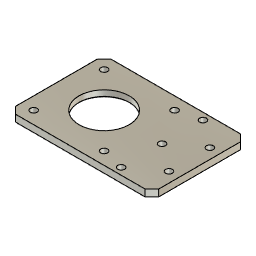
_机械臂组装 v14 (Autodesk Fusion 360 archive; units mm, degrees)
design "42电机输出固定"
Autodesk Fusion 360 part; units mm, degrees
(part 1 of 3)
sketch "草图1" plane through (0, 0, 0) normal (0, 0, 1) x (1, 0, 0)
  circle A0 centre (0, 0) radius 11.025
  line L0 (18, 21) -> (-18, 21)
  line L1 (-21, 18) -> (-21, -18)
  line L2 (-18, -21) -> (18, -21)
  line L3 (21, -18) -> (21, 18)
  line L4 (21, 21) -> (-21, -21) construction
  line L5 (-21, 21) -> (21, -21) construction
  circle A1 centre (15.5, -15.5) radius 1.5
  circle A2 centre (15.5, 15.5) radius 1.5
  circle A3 centre (-15.5, 15.5) radius 1.5
  circle A4 centre (-15.5, -15.5) radius 1.5
  line L6 (-18, 21) -> (-21, 18)
  line L7 (-21, -18) -> (-18, -21)
  line L8 (18, 21) -> (21, 18)
  line L9 (21, -18) -> (18, -21)
  line L10 (42, 18) -> (42, -18)
  line L11 (21, -18) -> (21, 18)
  line L12 (18, 21) -> (39, 21)
  line L13 (39, -21) -> (18, -21)
  circle A5 centre (25.5, 0) radius 1.5
  circle A6 centre (25.5, -18) radius 1.5
  circle A7 centre (37.5, -9) radius 1.5
  line L14 (79.2108, 0) -> (-40, 0) construction
  circle A8 centre (37.5, 9) radius 1.5
  circle A9 centre (25.5, 18) radius 1.5
  line L15 (39, 21) -> (42, 18)
  line L16 (42, -18) -> (39, -21)
  point P0 (42, 21)
  point P1 (42, -21)
  dimension "d1" = 22.05
  dimension "d2" = 42
  dimension "d3" = 42
  dimension "d4" = 15.5
  dimension "d5" = 3
  dimension "d7" = 360
  dimension "d8" = 3
  dimension "d9" = 3
  dimension "d10" = 3
  dimension "d11" = 3
  dimension "d12" = 3
  dimension "d13" = 3
  dimension "d14" = 3
  dimension "d15" = 3
  dimension "d17" = 21
  dimension "d20" = 3
  dimension "d21" = 3
  dimension "d22" = 3
  dimension "d24" = 18
  dimension "d25" = 9
  dimension "d26" = 4.5
  dimension "d27" = 4.5
  dimension "d28" = 16.5
  dimension "d30" = 3
  dimension "d31" = 3
  dimension "d32" = 3
  dimension "d33" = 3
  constraint coincident A0.centre origin
  constraint horizontal L0
  constraint perpendicular L0 L1
  constraint parallel L0 L2
  constraint parallel L1 L3
  constraint coincident L4 A0.centre
  constraint coincident L5 A0.centre
  constraint coincident L5 A1.centre
  constraint coincident L5.start L0
  constraint coincident L5.start L1
  constraint coincident L4.end L1
  constraint coincident L4.end L2
  constraint coincident L4.start L0
  constraint coincident L4.start L3
  constraint coincident L5.end L3
  constraint coincident L5.end L2
  constraint vertical L10
  constraint vertical L11
  constraint horizontal L12
  constraint horizontal L13
  constraint horizontal L14
  constraint coincident A0.centre L14
  constraint coincident A5.centre L14
  constraint symmetric A6 L14 A9
  constraint symmetric A7 L14 A8
  constraint coincident P0 L12
  constraint coincident P0 L10
  constraint coincident P1 L10
  constraint coincident P1 L13
  measures "d1" diameter of A0
  measures "d2" distance of L4.start L5.start
  measures "d3" distance of L4.start L5.end
  measures "d4" horizontal distance of A0.centre A1.centre
  measures "d5" diameter of A1
  measures "d8" distance of L5.start L0.end
  measures "d9" distance of L5.start L1.start
  measures "d10" distance of L4.end L1.end
  measures "d11" distance of L4.end L2.start
  measures "d12" distance of L4.start L0.start
  measures "d13" distance of L4.start L3.end
  measures "d14" distance of L5.end L3.start
  measures "d15" distance of L5.end L2.end
  measures "d17" distance of L10 L11
  measures "d20" diameter of A6
  measures "d21" diameter of A5
  measures "d22" diameter of A7
  measures "d24" distance of A6.centre L14
  measures "d25" distance of A7.centre L14
  measures "d26" distance of L11 A5.centre
  measures "d27" distance of L11 A6.centre
  measures "d28" distance of L3 A7.centre
  measures "d30" distance of P0 L12.end
  measures "d31" distance of P0 L10.start
  measures "d32" distance of P1 L10.end
  measures "d33" distance of P1 L13.start
extrude "拉伸1" add sketch "草图1" along normal blind 3
chamfer "倒角1" distance 0.5 angle 45 1 edges at (-10.2789, 3.9868, 0)
equation "d9 = d8"
equation "d11 = d10"
equation "d13 = d12"
equation "d15 = d14"
equation "d31 = d30"
equation "d33 = d32"

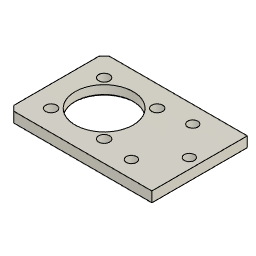
design "28减速输出固定"
Autodesk Fusion 360 part; units mm, degrees
sketch "草图4" plane through (0, 0, 0) normal (0, 0, 1) x (1, 0, 0)
  line L0 (12.5, 14) -> (-12.5, 14)
  line L1 (-14, 12.5) -> (-14, -12.5)
  line L2 (-12.5, -14) -> (12.5, -14)
  line L3 (14, -12.5) -> (14, 12.5)
  line L4 (14, 14) -> (-14, -14) construction
  line L5 (-14, 14) -> (14, -14) construction
  line L6 (12.5, 14) -> (14, 12.5)
  line L7 (14, -12.5) -> (12.5, -14)
  line L8 (-12.5, -14) -> (-14, -12.5)
  line L9 (-14, 12.5) -> (-12.5, 14)
  circle A0 centre (7.7782, 7.7782) radius 1.609
  circle A1 centre (0, 0) radius 8.5
  circle A2 centre (-7.7782, 7.7782) radius 1.609
  circle A3 centre (-7.7782, -7.7782) radius 1.609
  circle A4 centre (7.7782, -7.7782) radius 1.609
  line L10 (0, -35) -> (0, 45.3825) construction
  line L11 (12.5, 14) -> (28, 14)
  line L12 (28, 14) -> (28, -14)
  line L13 (28, -14) -> (12.5, -14)
  line L14 (-31, 0) -> (62, 0) construction
  circle A5 centre (25, 0) radius 1.5
  circle A6 centre (17, -9) radius 1.5
  circle A7 centre (17, 9) radius 1.5
  dimension "d49" = 28
  dimension "d50" = 28
  dimension "d51" = 1.5
  dimension "d52" = 1.5
  dimension "d53" = 1.5
  dimension "d54" = 1.5
  dimension "d55" = 1.5
  dimension "d56" = 1.5
  dimension "d57" = 1.5
  dimension "d58" = 1.5
  dimension "d59" = 11
  dimension "d60" = 17
  dimension "d62" = 360
  dimension "d71" = 14
  dimension "d72" = 3
  dimension "d73" = 3
  dimension "d74" = 3
  dimension "d75" = 11
  dimension "d76" = 9
  constraint horizontal L0
  constraint perpendicular L0 L1
  constraint parallel L0 L2
  constraint parallel L1 L3
  constraint coincident L4 A1.centre
  constraint coincident L5 A1.centre
  constraint coincident A1.centre origin
  constraint coincident L4.start L0
  constraint coincident L4.start L3
  constraint coincident L5.end L3
  constraint coincident L5.end L2
  constraint coincident L4.end L2
  constraint coincident L4.end L1
  constraint coincident L5.start L1
  constraint coincident L5.start L0
  constraint coincident L4 A0.centre
  constraint vertical L10
  constraint coincident A1.centre L10
  constraint parallel L0 L11
  constraint perpendicular L0 L12
  constraint horizontal L13
  constraint horizontal L14
  constraint coincident A1.centre L14
  constraint coincident L14 A5.centre
  constraint symmetric L14 A6 A7
  measures "d49" distance of L4.start L5.start
  measures "d50" distance of L5.start L4.end
  measures "d51" distance of L4.start L0.start
  measures "d52" distance of L4.start L3.end
  measures "d53" distance of L5.end L3.start
  measures "d54" distance of L5.end L2.end
  measures "d55" distance of L4.end L2.start
  measures "d56" distance of L4.end L1.end
  measures "d57" distance of L5.start L1.start
  measures "d58" distance of L5.start L0.end
  measures "d59" distance of A1.centre A0.centre
  measures "d60" diameter of A1
  measures "d71" distance of L3 L12
  measures "d72" diameter of A6
  measures "d73" diameter of A5
  measures "d74" distance of L3 A6.centre
  measures "d75" distance of L3 A5.centre
  measures "d76" distance of L14 A6.centre
extrude "拉伸3" add sketch "草图4" along normal blind 3
chamfer "倒角2" distance 0.5 angle 45 1 edges at (-7.9248, 3.0737, 0)
equation "d52 = d51"
equation "d54 = d53"
equation "d56 = d55"
equation "d58 = d57"

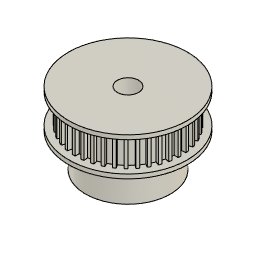
design "2GT40同步轮"
Autodesk Fusion 360 part; units mm, degrees
sketch "草图1" plane through (0, 0, 0) normal (0, 0, 1) x (1, 0, 0)
  circle A0 centre (0, 0) radius 10
  circle A1 centre (0, 0) radius 2.5
  dimension "d1" = 20
  dimension "d2" = 5
  constraint coincident A0.centre A1.centre
  measures "d1" diameter of A0
  measures "d2" diameter of A1
extrude "拉伸1" add sketch "草图1" along normal blind 8
sketch "草图2" plane through (0, 0, 0) normal (0, 0, 1) x (1, 0, 0)
  circle A0 centre (0, 0) radius 14
  line L0 (0, 0) -> (1.9515, 12.3214) construction
  line L1 (0, 0) -> (0, 12.475) construction
  line L2 (1.9501, 12.3124) -> (1.799, 11.3584)
  line L3 (1.799, 11.3584) -> (0.6019, 11.4842)
  line L4 (0.6529, 12.4579) -> (0, 12.4659)
  line L5 (0.6529, 12.4579) -> (0, 0) construction
  line L6 (0.6529, 12.4579) -> (0.6019, 11.4842)
  line L7 (0.6529, 12.4579) -> (0.6019, 11.4842)
  line L8 (-1.304, 12.4067) -> (-1.9501, 12.3124)
  line L9 (-1.304, 12.4067) -> (-1.2021, 11.437)
  line L10 (0, 11.5) -> (-1.2021, 11.437)
  line L11 (0, 12.4659) -> (0, 11.5)
  line L12 (-3.2288, 12.0499) -> (-3.8522, 11.8557)
  line L13 (-3.2288, 12.0499) -> (-2.9764, 11.1081)
  line L14 (-1.799, 11.3584) -> (-2.9764, 11.1081)
  line L15 (-1.9501, 12.3124) -> (-1.799, 11.3584)
  line L16 (-5.074, 11.3965) -> (-5.6594, 11.1072)
  line L17 (-5.074, 11.3965) -> (-4.6775, 10.5058)
  line L18 (-3.5537, 10.9371) -> (-4.6775, 10.5058)
  line L19 (-3.8522, 11.8557) -> (-3.5537, 10.9371)
  line L20 (-6.7944, 10.4624) -> (-7.3272, 10.0851)
  line L21 (-6.7944, 10.4624) -> (-6.2633, 9.6447)
  line L22 (-5.2209, 10.2466) -> (-6.2633, 9.6447)
  line L23 (-5.6594, 11.1072) -> (-5.2209, 10.2466)
  line L24 (-8.3474, 9.2707) -> (-8.8147, 8.8147)
  line L25 (-8.3474, 9.2707) -> (-7.695, 8.5462)
  line L26 (-6.7595, 9.3037) -> (-7.695, 8.5462)
  line L27 (-7.3272, 10.0851) -> (-6.7595, 9.3037)
  line L28 (-9.6949, 7.8508) -> (-10.0851, 7.3272)
  line L29 (-9.6949, 7.8508) -> (-8.9372, 7.2372)
  line L30 (-8.1317, 8.1317) -> (-8.9372, 7.2372)
  line L31 (-8.8147, 8.8147) -> (-8.1317, 8.1317)
  line L32 (-10.8037, 6.2375) -> (-11.1072, 5.6594)
  line L33 (-10.8037, 6.2375) -> (-9.9593, 5.75)
  line L34 (-9.3037, 6.7595) -> (-9.9593, 5.75)
  line L35 (-10.0851, 7.3272) -> (-9.3037, 6.7595)
  line L36 (-11.6464, 4.4706) -> (-11.8557, 3.8522)
  line L37 (-11.6464, 4.4706) -> (-10.7362, 4.1212)
  line L38 (-10.2466, 5.2209) -> (-10.7362, 4.1212)
  line L39 (-11.1072, 5.6594) -> (-10.2466, 5.2209)
  line L40 (-12.2024, 2.5937) -> (-12.3124, 1.9501)
  line L41 (-12.2024, 2.5937) -> (-11.2487, 2.391)
  line L42 (-10.9371, 3.5537) -> (-11.2487, 2.391)
  line L43 (-11.8557, 3.8522) -> (-10.9371, 3.5537)
  line L44 (-12.4579, 0.6529) -> (-12.4659, 0)
  line L45 (-12.4579, 0.6529) -> (-11.4842, 0.6019)
  line L46 (-11.3584, 1.799) -> (-11.4842, 0.6019)
  line L47 (-12.3124, 1.9501) -> (-11.3584, 1.799)
  line L48 (-12.4067, -1.304) -> (-12.3124, -1.9501)
  line L49 (-12.4067, -1.304) -> (-11.437, -1.2021)
  line L50 (-11.5, 0) -> (-11.437, -1.2021)
  line L51 (-12.4659, 0) -> (-11.5, 0)
  line L52 (-12.0499, -3.2288) -> (-11.8557, -3.8522)
  line L53 (-12.0499, -3.2288) -> (-11.1081, -2.9764)
  line L54 (-11.3584, -1.799) -> (-11.1081, -2.9764)
  line L55 (-12.3124, -1.9501) -> (-11.3584, -1.799)
  line L56 (-11.3965, -5.074) -> (-11.1072, -5.6594)
  line L57 (-11.3965, -5.074) -> (-10.5058, -4.6775)
  line L58 (-10.9371, -3.5537) -> (-10.5058, -4.6775)
  line L59 (-11.8557, -3.8522) -> (-10.9371, -3.5537)
  line L60 (-10.4624, -6.7944) -> (-10.0851, -7.3272)
  line L61 (-10.4624, -6.7944) -> (-9.6447, -6.2633)
  line L62 (-10.2466, -5.2209) -> (-9.6447, -6.2633)
  line L63 (-11.1072, -5.6594) -> (-10.2466, -5.2209)
  line L64 (-9.2707, -8.3474) -> (-8.8147, -8.8147)
  line L65 (-9.2707, -8.3474) -> (-8.5462, -7.695)
  line L66 (-9.3037, -6.7595) -> (-8.5462, -7.695)
  line L67 (-10.0851, -7.3272) -> (-9.3037, -6.7595)
  line L68 (-7.8508, -9.6949) -> (-7.3272, -10.0851)
  line L69 (-7.8508, -9.6949) -> (-7.2372, -8.9372)
  line L70 (-8.1317, -8.1317) -> (-7.2372, -8.9372)
  line L71 (-8.8147, -8.8147) -> (-8.1317, -8.1317)
  line L72 (-6.2375, -10.8037) -> (-5.6594, -11.1072)
  line L73 (-6.2375, -10.8037) -> (-5.75, -9.9593)
  line L74 (-6.7595, -9.3037) -> (-5.75, -9.9593)
  line L75 (-7.3272, -10.0851) -> (-6.7595, -9.3037)
  line L76 (-4.4706, -11.6464) -> (-3.8522, -11.8557)
  line L77 (-4.4706, -11.6464) -> (-4.1212, -10.7362)
  line L78 (-5.2209, -10.2466) -> (-4.1212, -10.7362)
  line L79 (-5.6594, -11.1072) -> (-5.2209, -10.2466)
  line L80 (-2.5937, -12.2024) -> (-1.9501, -12.3124)
  line L81 (-2.5937, -12.2024) -> (-2.391, -11.2487)
  line L82 (-3.5537, -10.9371) -> (-2.391, -11.2487)
  line L83 (-3.8522, -11.8557) -> (-3.5537, -10.9371)
  line L84 (-0.6529, -12.4579) -> (0, -12.4659)
  line L85 (-0.6529, -12.4579) -> (-0.6019, -11.4842)
  line L86 (-1.799, -11.3584) -> (-0.6019, -11.4842)
  line L87 (-1.9501, -12.3124) -> (-1.799, -11.3584)
  line L88 (1.304, -12.4067) -> (1.9501, -12.3124)
  line L89 (1.304, -12.4067) -> (1.2021, -11.437)
  line L90 (0, -11.5) -> (1.2021, -11.437)
  line L91 (0, -12.4659) -> (0, -11.5)
  line L92 (3.2288, -12.0499) -> (3.8522, -11.8557)
  line L93 (3.2288, -12.0499) -> (2.9764, -11.1081)
  line L94 (1.799, -11.3584) -> (2.9764, -11.1081)
  line L95 (1.9501, -12.3124) -> (1.799, -11.3584)
  line L96 (5.074, -11.3965) -> (5.6594, -11.1072)
  line L97 (5.074, -11.3965) -> (4.6775, -10.5058)
  line L98 (3.5537, -10.9371) -> (4.6775, -10.5058)
  line L99 (3.8522, -11.8557) -> (3.5537, -10.9371)
  line L100 (6.7944, -10.4624) -> (7.3272, -10.0851)
  line L101 (6.7944, -10.4624) -> (6.2633, -9.6447)
  line L102 (5.2209, -10.2466) -> (6.2633, -9.6447)
  line L103 (5.6594, -11.1072) -> (5.2209, -10.2466)
  line L104 (8.3474, -9.2707) -> (8.8147, -8.8147)
  line L105 (8.3474, -9.2707) -> (7.695, -8.5462)
  line L106 (6.7595, -9.3037) -> (7.695, -8.5462)
  line L107 (7.3272, -10.0851) -> (6.7595, -9.3037)
  line L108 (9.6949, -7.8508) -> (10.0851, -7.3272)
  line L109 (9.6949, -7.8508) -> (8.9372, -7.2372)
  line L110 (8.1317, -8.1317) -> (8.9372, -7.2372)
  line L111 (8.8147, -8.8147) -> (8.1317, -8.1317)
  line L112 (10.8037, -6.2375) -> (11.1072, -5.6594)
  line L113 (10.8037, -6.2375) -> (9.9593, -5.75)
  line L114 (9.3037, -6.7595) -> (9.9593, -5.75)
  line L115 (10.0851, -7.3272) -> (9.3037, -6.7595)
  line L116 (11.6464, -4.4706) -> (11.8557, -3.8522)
  line L117 (11.6464, -4.4706) -> (10.7362, -4.1212)
  line L118 (10.2466, -5.2209) -> (10.7362, -4.1212)
  line L119 (11.1072, -5.6594) -> (10.2466, -5.2209)
  line L120 (12.2024, -2.5937) -> (12.3124, -1.9501)
  line L121 (12.2024, -2.5937) -> (11.2487, -2.391)
  line L122 (10.9371, -3.5537) -> (11.2487, -2.391)
  line L123 (11.8557, -3.8522) -> (10.9371, -3.5537)
  line L124 (12.4579, -0.6529) -> (12.4659, 0)
  line L125 (12.4579, -0.6529) -> (11.4842, -0.6019)
  line L126 (11.3584, -1.799) -> (11.4842, -0.6019)
  line L127 (12.3124, -1.9501) -> (11.3584, -1.799)
  line L128 (12.4067, 1.304) -> (12.3124, 1.9501)
  line L129 (12.4067, 1.304) -> (11.437, 1.2021)
  line L130 (11.5, 0) -> (11.437, 1.2021)
  line L131 (12.4659, 0) -> (11.5, 0)
  line L132 (12.0499, 3.2288) -> (11.8557, 3.8522)
  line L133 (12.0499, 3.2288) -> (11.1081, 2.9764)
  line L134 (11.3584, 1.799) -> (11.1081, 2.9764)
  line L135 (12.3124, 1.9501) -> (11.3584, 1.799)
  line L136 (11.3965, 5.074) -> (11.1072, 5.6594)
  line L137 (11.3965, 5.074) -> (10.5058, 4.6775)
  line L138 (10.9371, 3.5537) -> (10.5058, 4.6775)
  line L139 (11.8557, 3.8522) -> (10.9371, 3.5537)
  line L140 (10.4624, 6.7944) -> (10.0851, 7.3272)
  line L141 (10.4624, 6.7944) -> (9.6447, 6.2633)
  line L142 (10.2466, 5.2209) -> (9.6447, 6.2633)
  line L143 (11.1072, 5.6594) -> (10.2466, 5.2209)
  line L144 (9.2707, 8.3474) -> (8.8147, 8.8147)
  line L145 (9.2707, 8.3474) -> (8.5462, 7.695)
  line L146 (9.3037, 6.7595) -> (8.5462, 7.695)
  line L147 (10.0851, 7.3272) -> (9.3037, 6.7595)
  line L148 (7.8508, 9.6949) -> (7.3272, 10.0851)
  line L149 (7.8508, 9.6949) -> (7.2372, 8.9372)
  line L150 (8.1317, 8.1317) -> (7.2372, 8.9372)
  line L151 (8.8147, 8.8147) -> (8.1317, 8.1317)
  line L152 (6.2375, 10.8037) -> (5.6594, 11.1072)
  line L153 (6.2375, 10.8037) -> (5.75, 9.9593)
  line L154 (6.7595, 9.3037) -> (5.75, 9.9593)
  line L155 (7.3272, 10.0851) -> (6.7595, 9.3037)
  line L156 (4.4706, 11.6464) -> (3.8522, 11.8557)
  line L157 (4.4706, 11.6464) -> (4.1212, 10.7362)
  line L158 (5.2209, 10.2466) -> (4.1212, 10.7362)
  line L159 (5.6594, 11.1072) -> (5.2209, 10.2466)
  line L160 (2.5937, 12.2024) -> (1.9501, 12.3124)
  line L161 (2.5937, 12.2024) -> (2.391, 11.2487)
  line L162 (3.5537, 10.9371) -> (2.391, 11.2487)
  line L163 (3.8522, 11.8557) -> (3.5537, 10.9371)
  circle A1 centre (0, 0) radius 2.5
  dimension "d5" = 28
  dimension "d6" = 9
  dimension "d7" = 12.475
  dimension "d12" = 360
  dimension "d16" = 11.5
  dimension "d17" = 11.5
  dimension "d19" = 3
  dimension "d23" = 5
  constraint coincident A0.centre L0.start
  constraint vertical L1
  constraint coincident L0 L2.end
  constraint parallel L0 L2
  constraint coincident L5 L3.end
  constraint equal L1 L5
  constraint equal L0 L1
  measures "d5" diameter of A0
  measures "d6" angle of L0 L1
  measures "d7" distance of A0.centre L1.end
  measures "d16" distance of A0.centre L3.end
  measures "d17" distance of A0.centre L2.end
  measures "d19" angle of L1 L6
  measures "d23" diameter of A1
extrude "拉伸2" add sketch "草图2" along normal blind 9 from surface at 8 contours A0 | L2 L3 L4 L6 L7 L8 L9 L10 L11 L12 L13 L14 L15 L16 L17 L18 L19 L20 L21 L22 L23 L24 L25 L26 L27 L28 L29 L30 L31 L32 L33 L34 L35 L36 L37 L38 L39 L40 L41 L42 L43 L44 L45 L46 L47 L48 L49 L50 L51 L52 L53 L54 L55 L56 L57 L58 L59 L60 L61 L62 L63 L64 L65 L66 L67 L68 L69 L70 L71 L72 L73 L74 L75 L76 L77 L78 L79 L80 L81 L82 L83 L84 L85 L86 L87 L88 L89 L90 L91 L92 L93 L94 L95 L96 L97 L98 L99 L100 L101 L102 L103 L104 L105 L106 L107 L108 L109 L110 L111 L112 L113 L114 L115 L116 L117 L118 L119 L120 L121 L122 L123 L124 L125 L126 L127 L128 L129 L130 L131 L132 L133 L134 L135 L136 L137 L138 L139 L140 L141 L142 L143 L144 L145 L146 L147 L148 L149 L150 L151 L152 L153 L154 L155 L156 L157 L158 L159 L160 L161 L162 L163
extrude "拉伸3" cut sketch "草图2" along normal blind 7 from surface at 9 contours A0

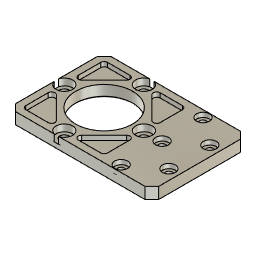
design "42减速输出固定"
Autodesk Fusion 360 part; units mm, degrees
sketch "草图1" plane through (0, 0, 0) normal (0, 0, 1) x (1, 0, 0)
  circle A0 centre (0, 0) radius 12.525
  line L0 (18, 21) -> (-18, 21)
  line L1 (-21, 18) -> (-21, -18)
  line L2 (-18, -21) -> (18, -21)
  line L3 (21, -18) -> (21, 18)
  line L4 (21, 21) -> (-21, -21) construction
  line L5 (-21, 21) -> (21, -21) construction
  line L6 (-18, 21) -> (-21, 18)
  line L7 (-21, -18) -> (-18, -21)
  line L8 (18, -21) -> (21, -18)
  line L9 (21, 18) -> (18, 21)
  line L10 (18, 21) -> (39, 21)
  line L11 (42, 18) -> (42, -18)
  line L12 (39, -21) -> (18, -21)
  circle A1 centre (0, 17.5) radius 2
  line L13 (0, 43) -> (0, -30.7766) construction
  circle A2 centre (-17.5, 0) radius 2
  circle A3 centre (0, -17.5) radius 2
  circle A4 centre (17.5, 0) radius 2
  circle A5 centre (37.5, 9) radius 1.5
  circle A6 centre (25.5, 0) radius 1.5
  circle A7 centre (37.5, -9) radius 1.5
  circle A8 centre (25.5, -18) radius 1.5
  circle A9 centre (25.5, 18) radius 1.5
  line L14 (-27.6866, 0) -> (52.7849, 0) construction
  line L15 (39, 21) -> (42, 18)
  line L16 (42, -18) -> (39, -21)
  point P0 (42, 21)
  point P1 (42, -21)
  dimension "d1" = 25.05
  dimension "d2" = 42
  dimension "d3" = 42
  dimension "d4" = 3
  dimension "d5" = 3
  dimension "d6" = 3
  dimension "d7" = 3
  dimension "d8" = 3
  dimension "d9" = 3
  dimension "d10" = 3
  dimension "d11" = 3
  dimension "d12" = 21
  dimension "d13" = 4
  dimension "d14" = 17.5
  dimension "d16" = 360
  dimension "d20" = 3
  dimension "d21" = 3
  dimension "d22" = 3
  dimension "d23" = 4.5
  dimension "d24" = 16.5
  dimension "d25" = 18
  dimension "d26" = 9
  dimension "d28" = 4.5
  dimension "d49" = 3
  dimension "d50" = 3
  dimension "d51" = 3
  dimension "d52" = 3
  constraint coincident A0.centre origin
  constraint horizontal L0
  constraint perpendicular L0 L1
  constraint parallel L0 L2
  constraint parallel L1 L3
  constraint coincident L4 A0.centre
  constraint coincident L5 A0.centre
  constraint coincident L5.start L0
  constraint coincident L5.start L1
  constraint coincident L4.end L1
  constraint coincident L4.end L2
  constraint coincident L5.end L2
  constraint coincident L5.end L3
  constraint coincident L4.start L3
  constraint coincident L4.start L0
  constraint parallel L0 L10
  constraint perpendicular L10 L11
  constraint perpendicular L2 L13
  constraint coincident A0.centre L13
  constraint coincident A1.centre L13
  constraint horizontal L14
  constraint coincident A0.centre L14
  constraint coincident A6.centre L14
  constraint symmetric A8 A9 L14
  constraint symmetric A5 A7 L14
  constraint horizontal L12
  constraint coincident P0 L10
  constraint coincident P0 L11
  constraint coincident P1 L11
  constraint coincident P1 L12
  measures "d1" diameter of A0
  measures "d2" distance of L4.start L5.end
  measures "d3" distance of L4.start L5.start
  measures "d4" distance of L5.start L0.end
  measures "d5" distance of L5.start L1.start
  measures "d6" distance of L4.end L1.end
  measures "d7" distance of L4.end L2.start
  measures "d8" distance of L5.end L2.end
  measures "d9" distance of L5.end L3.start
  measures "d10" distance of L4.start L3.end
  measures "d11" distance of L4.start L0.start
  measures "d12" distance of L3 L11
  measures "d13" diameter of A1
  measures "d14" distance of A0.centre A1.centre
  measures "d20" diameter of A8
  measures "d21" diameter of A6
  measures "d22" diameter of A7
  measures "d23" distance of L3 A6.centre
  measures "d24" distance of L3 A7.centre
  measures "d25" distance of A8.centre L14
  measures "d26" distance of A7.centre L14
  measures "d28" distance of L3 A8.centre
  measures "d49" distance of P0 L10.end
  measures "d50" distance of P0 L11.start
  measures "d51" distance of P1 L11.end
  measures "d52" distance of P1 L12.start
extrude "拉伸1" add sketch "草图1" along normal blind 5
sketch "草图2" plane through (0, 0, 5) normal (0, 0, 1) x (-1, 0, 0)
  circle A0 centre (-17.5, 0) radius 2
  circle A1 centre (0, -17.5) radius 2
  circle A2 centre (17.5, 0) radius 2
  circle A3 centre (0, 17.5) radius 2
  circle A4 centre (0, 0) radius 12.525
  circle A5 centre (-37.5, -9) radius 1.5
  circle A6 centre (-25.5, 0) radius 1.5
  circle A7 centre (-37.5, 9) radius 1.5
  circle A8 centre (-25.5, 18) radius 1.5
  circle A9 centre (-25.5, -18) radius 1.5
  line L0 (-39, -21) -> (18, -21)
  line L1 (18, -21) -> (21, -18)
  line L2 (21, -18) -> (21, 18)
  line L3 (21, 18) -> (18, 21)
  line L4 (18, 21) -> (-39, 21)
  line L5 (-42, 18) -> (-42, -18)
  circle A10 centre (0, -17.5) radius 2
  circle A11 centre (-25.5, 0) radius 1.5
  circle A12 centre (-37.5, -9) radius 1.5
  circle A13 centre (-25.5, -18) radius 1.5
  circle A14 centre (-37.5, 9) radius 1.5
  circle A15 centre (-25.5, 18) radius 1.5
  circle A16 centre (0, 17.5) radius 2
  circle A17 centre (-17.5, 0) radius 2
  circle A18 centre (17.5, 0) radius 2
  line L6 (-39, 21) -> (-42, 18)
  line L7 (-42, -18) -> (-39, -21)
  constraint concentric A1 A10
  constraint concentric A6 A11
  constraint concentric A5 A12
  constraint concentric A9 A13
  constraint concentric A7 A14
  constraint concentric A8 A15
  constraint concentric A3 A16
  constraint concentric A0 A17
  constraint concentric A2 A18
hole "孔1" at (-17.5, 0, 5) at (0, 17.5, 5) at (17.5, 0, 5) at (0, -17.5, 5) direction (0, 0, -1) diameter 4 depth 13 tip angle 180 counterbore diameter 7.25 counterbore depth 3
hole "孔2" at (25.5, 0, 5) at (37.5, 9, 5) at (25.5, 18, 5) at (37.5, -9, 5) at (25.5, -18, 5) direction (0, 0, -1) diameter 3 depth 13 tip angle 180 counterbore diameter 5.7 counterbore depth 2
chamfer "倒角1" distance 0.5 angle 45 1 edges at (-11.6774, 4.5292, 0)
sketch "草图3" plane through (0, 0, 0) normal (0, 0, 1) x (1, 0, 0)
  line L0 (-16.5, 18) -> (-6.6213, 18)
  line L1 (-5.5607, 15.4393) -> (-15.4393, 5.5607)
  line L2 (-18, 6.6213) -> (-18, 16.5)
  arc A0 (-5.5607, 15.4393) -> (-6.6213, 18) centre (-6.6213, 16.5) ccw
  arc A1 (-18, 6.6213) -> (-15.4393, 5.5607) centre (-16.5, 6.6213) ccw
  arc A2 (-16.5, 18) -> (-18, 16.5) centre (-16.5, 16.5) ccw
  line L3 (-18, -16.5) -> (-18, -6.6213)
  arc A3 (-15.4393, -5.5607) -> (-18, -6.6213) centre (-16.5, -6.6213) ccw
  line L4 (-15.4393, -5.5607) -> (-5.5607, -15.4393)
  arc A4 (-6.6213, -18) -> (-5.5607, -15.4393) centre (-6.6213, -16.5) ccw
  line L5 (-6.6213, -18) -> (-16.5, -18)
  arc A5 (-18, -16.5) -> (-16.5, -18) centre (-16.5, -16.5) ccw
  line L6 (16.5, -18) -> (6.6213, -18)
  arc A6 (5.5607, -15.4393) -> (6.6213, -18) centre (6.6213, -16.5) ccw
  line L7 (5.5607, -15.4393) -> (15.4393, -5.5607)
  arc A7 (18, -6.6213) -> (15.4393, -5.5607) centre (16.5, -6.6213) ccw
  line L8 (18, -6.6213) -> (18, -16.5)
  arc A8 (16.5, -18) -> (18, -16.5) centre (16.5, -16.5) ccw
  line L9 (18, 16.5) -> (18, 6.6213)
  arc A9 (15.4393, 5.5607) -> (18, 6.6213) centre (16.5, 6.6213) ccw
  line L10 (15.4393, 5.5607) -> (5.5607, 15.4393)
  arc A10 (6.6213, 18) -> (5.5607, 15.4393) centre (6.6213, 16.5) ccw
  line L11 (6.6213, 18) -> (16.5, 18)
  arc A11 (18, 16.5) -> (16.5, 18) centre (16.5, 16.5) ccw
  point P0 (-18, 18)
  point P1 (-3, 18)
  dimension "d40" = 18
  dimension "d41" = 18
  dimension "d42" = 15
  dimension "d43" = 1.5
  dimension "d45" = 360
  constraint horizontal L0
  constraint vertical L2
  constraint coincident P1 L0
  constraint coincident P1 L1
  constraint tangent L0 A0
  constraint tangent L1 A0
  constraint tangent L1 A1
  constraint tangent L2 A1
  constraint equal A0 A1
  constraint coincident P0 L2
  constraint coincident P0 L0
  constraint tangent L2 A2
  constraint tangent L0 A2
  constraint equal A0 A2
  constraint equal L0 L2
  measures "d40" distance of origin L0
  measures "d41" distance of origin L2
  measures "d42" distance of P0 P1
  measures "d43" radius of A0
extrude "拉伸2" cut sketch "草图3" against normal blind 2 from surface at 5
equation "d5 = d4"
equation "d7 = d6"
equation "d9 = d8"
equation "d11 = d10"
equation "d50 = d49"
equation "d52 = d51"

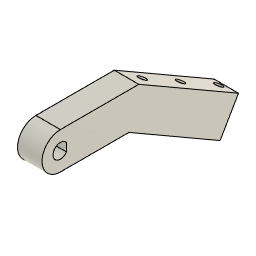
design "28输出Joint-4"
Autodesk Fusion 360 part; units mm, degrees
sketch "草图1" plane through (0, 0, 0) normal (1, 0, 0) x (0, 1, 0)
  circle A0 centre (0, 0) radius 7.5
  line L0 (0, 7.5) -> (32.0096, 7.5)
  line L1 (32.0096, 7.5) -> (72.7211, -16.0048)
  line L2 (72.7211, -16.0048) -> (65.2211, -28.9952)
  line L3 (65.2211, -28.9952) -> (27.9904, -7.5)
  line L4 (27.9904, -7.5) -> (0, -7.5)
  line L5 (0, 0) -> (30, 0) construction
  line L6 (30, 0) -> (68.9711, -22.5) construction
  line L7 (2.5, 1.6583) -> (2.5, -1.6583)
  arc A1 (2.5, 1.6583) -> (2.5, -1.6583) centre (0, 0) ccw
  dimension "d1" = 6
  dimension "d2" = 15
  dimension "d4" = 15
  dimension "d5" = 150
  dimension "d7" = 45
  dimension "d8" = 30
  dimension "d11" = 2.5
  constraint coincident A0.centre L5.start
  constraint concentric A0 A1
  constraint coincident A0 L0.start
  constraint tangent A0 L0
  constraint horizontal L0
  constraint parallel L1 L3
  constraint parallel L0 L4
  constraint coincident A0 L4.end
  constraint tangent A0 L4
  constraint perpendicular L1 L2
  constraint parallel L4 L5
  constraint midpoint L2 L6.end
  constraint parallel L1 L6
  constraint vertical L7
  measures "d1" diameter of A1
  measures "d2" diameter of A0
  measures "d4" distance of L1.end L2.end
  measures "d5" angle of L3 L4
  measures "d7" distance of L5.end L6.end
  measures "d8" distance of A0.centre L5.end
  measures "d11" distance of A0.centre L7
extrude "拉伸1" add sketch "草图1" along normal blind 10
sketch "草图2" plane through (0, 11.25, 19.4856) normal (0, 0.5, 0.866025) x (-1, 0, 0)
  line L0 (0, -70.9808) -> (0, -23.9711)
  line L1 (0, -23.9711) -> (-10, -23.9711)
  line L2 (-10, -23.9711) -> (-10, -70.9808)
  line L3 (-10, -70.9808) -> (0, -70.9808)
  line L4 (-23.5973, -49.9808) -> (11.4027, -49.9808) construction
  line L5 (-4.5, -11.5429) -> (-4.5, -79.5429) construction
  circle A0 centre (-4.5, -49.9808) radius 1.5
  circle A1 centre (-4.5, -67.9808) radius 1.5
  circle A2 centre (-4.5, -31.9808) radius 1.5
  dimension "d12" = 21
  dimension "d13" = 4.5
  dimension "d14" = 3
  dimension "d15" = 3
  dimension "d16" = 18
  constraint perpendicular L2 L4
  constraint parallel L2 L5
  constraint coincident L5 A0.centre
  constraint coincident L4 A0.centre
  constraint coincident L5 A1.centre
  constraint symmetric L4 A1 A2
  measures "d12" distance of L3 L4
  measures "d13" distance of L0 L5
  measures "d14" diameter of A1
  measures "d15" diameter of A0
  measures "d16" distance of L4 A1.centre
hole "孔1" at (4.5, 70.1231, -14.5048) at (4.5, 54.5346, -5.5048) at (4.5, 38.9462, 3.4952) direction (0, -0.5, -0.866025) diameter 3.332 depth 10 tip angle 118
thread "螺纹1" "ISO Metric profile 4.0 M4x0.7 6H"

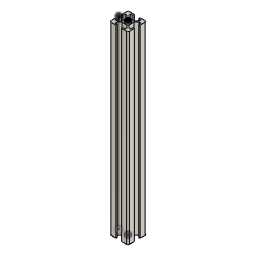
design "20*200铝型材"
Autodesk Fusion 360 part; units mm, degrees
sketch "草图1" plane through (0, 0, 0) normal (0, 0, 1) x (1, 0, 0)
  line L0 (8.5, 10) -> (-8.5, 10)
  line L1 (-10, 8.5) -> (-10, -8.5)
  line L2 (-8.5, -10) -> (8.5, -10)
  line L3 (10, -8.5) -> (10, 8.5)
  line L4 (10, 10) -> (-10, -10) construction
  line L5 (-10, 10) -> (10, -10) construction
  arc A0 (10, 8.5) -> (8.5, 10) centre (8.5, 8.5) ccw
  arc A1 (8.5, -10) -> (10, -8.5) centre (8.5, -8.5) ccw
  arc A2 (-10, -8.5) -> (-8.5, -10) centre (-8.5, -8.5) ccw
  arc A3 (-8.5, 10) -> (-10, 8.5) centre (-8.5, 8.5) ccw
  circle A4 centre (0, 0) radius 2.6
  line L6 (2.7393, 3.8) -> (5.5, 6.5607)
  line L7 (5.5, 6.5607) -> (5.5, 8.5)
  line L8 (5.5, 8.5) -> (3.15, 8.5)
  line L9 (3.15, 8.5) -> (3.15, 10)
  line L10 (2.7393, 3.8) -> (-2.7393, 3.8)
  line L11 (-2.7393, 3.8) -> (-5.5, 6.5607)
  line L12 (-5.5, 6.5607) -> (-5.5, 8.5)
  line L13 (-5.5, 8.5) -> (-3.15, 8.5)
  line L14 (-3.15, 8.5) -> (-3.15, 10)
  line L15 (0, 15.5) -> (0, 0)
  line L16 (-8.5, 3.15) -> (-10, 3.15)
  line L17 (-8.5, 5.5) -> (-8.5, 3.15)
  line L18 (-6.5607, 5.5) -> (-8.5, 5.5)
  line L19 (-3.8, 2.7393) -> (-6.5607, 5.5)
  line L20 (-3.8, 2.7393) -> (-3.8, -2.7393)
  line L21 (-3.8, -2.7393) -> (-6.5607, -5.5)
  line L22 (-6.5607, -5.5) -> (-8.5, -5.5)
  line L23 (-8.5, -5.5) -> (-8.5, -3.15)
  line L24 (-8.5, -3.15) -> (-10, -3.15)
  line L25 (-3.15, -8.5) -> (-3.15, -10)
  line L26 (-5.5, -8.5) -> (-3.15, -8.5)
  line L27 (-5.5, -6.5607) -> (-5.5, -8.5)
  line L28 (-2.7393, -3.8) -> (-5.5, -6.5607)
  line L29 (-2.7393, -3.8) -> (2.7393, -3.8)
  line L30 (2.7393, -3.8) -> (5.5, -6.5607)
  line L31 (5.5, -6.5607) -> (5.5, -8.5)
  line L32 (5.5, -8.5) -> (3.15, -8.5)
  line L33 (3.15, -8.5) -> (3.15, -10)
  line L34 (8.5, -3.15) -> (10, -3.15)
  line L35 (8.5, -5.5) -> (8.5, -3.15)
  line L36 (6.5607, -5.5) -> (8.5, -5.5)
  line L37 (3.8, -2.7393) -> (6.5607, -5.5)
  line L38 (3.8, -2.7393) -> (3.8, 2.7393)
  line L39 (3.8, 2.7393) -> (6.5607, 5.5)
  line L40 (6.5607, 5.5) -> (8.5, 5.5)
  line L41 (8.5, 5.5) -> (8.5, 3.15)
  line L42 (8.5, 3.15) -> (10, 3.15)
  dimension "d1" = 20
  dimension "d2" = 1.5
  dimension "d3" = 1.5
  dimension "d4" = 5.2
  dimension "d5" = 0.75
  dimension "d6" = 6.3
  dimension "d7" = 6.2
  dimension "d8" = 11
  dimension "d10" = 360
  dimension "d13" = 1.5
  constraint horizontal L0
  constraint perpendicular L0 L1
  constraint parallel L0 L2
  constraint parallel L1 L3
  constraint coincident L4 A4.centre
  constraint coincident L5 A4.centre
  constraint coincident A4.centre L15.end
  constraint coincident L4.start L0
  constraint coincident L4.start L3
  constraint tangent L0 A0
  constraint tangent L3 A0
  constraint coincident L5.end L3
  constraint coincident L5.end L2
  constraint tangent L3 A1
  constraint tangent L2 A1
  constraint coincident L4.end L1
  constraint coincident L4.end L2
  constraint tangent L1 A2
  constraint tangent L2 A2
  constraint equal A1 A2
  constraint coincident L5.start L1
  constraint coincident L5.start L0
  constraint tangent L1 A3
  constraint tangent L0 A3
  constraint equal A1 A3
  constraint parallel L4 L6
  constraint vertical L7
  constraint perpendicular L7 L8
  constraint coincident L0 L9.end
  constraint perpendicular L0 L9
  constraint horizontal L10
  constraint perpendicular L6 L11
  constraint vertical L12
  constraint perpendicular L12 L13
  constraint coincident L0 L14.end
  constraint perpendicular L0 L14
  constraint equal L6 L11
  constraint vertical L15
  constraint symmetric L9 L14 L15
  constraint symmetric L6 L11 L15
  constraint symmetric L7 L12 L15
  constraint symmetric L8 L13 L15
  measures "d1" distance of L4.start L5.start
  measures "d2" radius of A0
  measures "d3" radius of A1
  measures "d4" diameter of A4
  measures "d5" distance of L4 L6
  measures "d6" distance of L9 L14
  measures "d7" distance of L0 L10
  measures "d8" distance of L7 L12
  measures "d13" distance of L8.end L9.end
extrude "拉伸1" add sketch "草图1" along normal blind 200 contours L0 L1 L2 L3 A0 A1 A2 A3 L6 L7 L8 L9 L10 L11 L12 L13 L14 L16 L17 L18 L19 L20 L21 L22 L23 L24 L25 L26 L27 L28 L29 L30 L31 L32 L33 L34 L35 L36 L37 L38 L39 L40 L41 L42
ref_plane "工作平面1" through (-10, 0, 0) normal (1, 0, 0) x (0, 1, 0)
sketch "草图3" plane through (-10, 0, 0) normal (1, 0, 0) x (0, 1, 0)
  line L0 (0, 0) -> (0, 200)
  dimension "d15" = 200
  constraint vertical L0
  constraint coincident origin L0
  constraint coincident L0.start origin
  measures "d15" distance of L0.start L0.end
sketch "草图4" plane through (0, 0, 0) normal (0, 0, 1) x (1, 0, 0)
sketch "草图5" plane through (0, 0, 200) normal (0, 0, 1) x (-1, 0, 0)
  circle A0 centre (0, 0) radius 2.6
  line L0 (-3.8, 2.7393) -> (-3.8, -2.7393)
  line L1 (-3.8, -2.7393) -> (-6.5607, -5.5)
  line L2 (-6.5607, -5.5) -> (-8.5, -5.5)
  line L3 (-8.5, -5.5) -> (-8.5, -3.15)
  line L4 (-8.5, -3.15) -> (-10, -3.15)
  line L5 (-10, -3.15) -> (-10, -8.5)
  arc A1 (-10, -8.5) -> (-8.5, -10) centre (-8.5, -8.5) ccw
  line L6 (-8.5, -10) -> (-3.15, -10)
  line L7 (-3.15, -10) -> (-3.15, -8.5)
  line L8 (-3.15, -8.5) -> (-5.5, -8.5)
  line L9 (-5.5, -8.5) -> (-5.5, -6.5607)
  line L10 (-5.5, -6.5607) -> (-2.7393, -3.8)
  line L11 (-2.7393, -3.8) -> (2.7393, -3.8)
  line L12 (2.7393, -3.8) -> (5.5, -6.5607)
  line L13 (5.5, -6.5607) -> (5.5, -8.5)
  line L14 (5.5, -8.5) -> (3.15, -8.5)
  line L15 (3.15, -8.5) -> (3.15, -10)
  line L16 (3.15, -10) -> (8.5, -10)
  arc A2 (8.5, -10) -> (10, -8.5) centre (8.5, -8.5) ccw
  line L17 (10, -8.5) -> (10, -3.15)
  line L18 (10, -3.15) -> (8.5, -3.15)
  line L19 (8.5, -3.15) -> (8.5, -5.5)
  line L20 (8.5, -5.5) -> (6.5607, -5.5)
  line L21 (6.5607, -5.5) -> (3.8, -2.7393)
  line L22 (3.8, -2.7393) -> (3.8, 2.7393)
  line L23 (3.8, 2.7393) -> (6.5607, 5.5)
  line L24 (6.5607, 5.5) -> (8.5, 5.5)
  line L25 (8.5, 5.5) -> (8.5, 3.15)
  line L26 (8.5, 3.15) -> (10, 3.15)
  line L27 (10, 3.15) -> (10, 8.5)
  arc A3 (10, 8.5) -> (8.5, 10) centre (8.5, 8.5) ccw
  line L28 (8.5, 10) -> (3.15, 10)
  line L29 (3.15, 10) -> (3.15, 8.5)
  line L30 (3.15, 8.5) -> (5.5, 8.5)
  line L31 (5.5, 8.5) -> (5.5, 6.5607)
  line L32 (5.5, 6.5607) -> (2.7393, 3.8)
  line L33 (2.7393, 3.8) -> (-2.7393, 3.8)
  line L34 (-2.7393, 3.8) -> (-5.5, 6.5607)
  line L35 (-5.5, 6.5607) -> (-5.5, 8.5)
  line L36 (-5.5, 8.5) -> (-3.15, 8.5)
  line L37 (-3.15, 8.5) -> (-3.15, 10)
  line L38 (-3.15, 10) -> (-8.5, 10)
  arc A4 (-8.5, 10) -> (-10, 8.5) centre (-8.5, 8.5) ccw
  line L39 (-10, 8.5) -> (-10, 3.15)
  line L40 (-10, 3.15) -> (-8.5, 3.15)
  line L41 (-8.5, 3.15) -> (-8.5, 5.5)
  line L42 (-8.5, 5.5) -> (-6.5607, 5.5)
  line L43 (-6.5607, 5.5) -> (-3.8, 2.7393)
  constraint coincident A0.centre origin

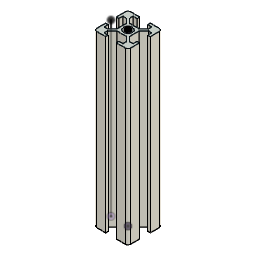
design "20*100铝型材"
Autodesk Fusion 360 part; units mm, degrees
sketch "草图1" plane through (0, 0, 0) normal (0, 0, 1) x (1, 0, 0)
  line L0 (8.5, 10) -> (-8.5, 10)
  line L1 (-10, 8.5) -> (-10, -8.5)
  line L2 (-8.5, -10) -> (8.5, -10)
  line L3 (10, -8.5) -> (10, 8.5)
  line L4 (10, 10) -> (-10, -10) construction
  line L5 (-10, 10) -> (10, -10) construction
  arc A0 (10, 8.5) -> (8.5, 10) centre (8.5, 8.5) ccw
  arc A1 (8.5, -10) -> (10, -8.5) centre (8.5, -8.5) ccw
  arc A2 (-10, -8.5) -> (-8.5, -10) centre (-8.5, -8.5) ccw
  arc A3 (-8.5, 10) -> (-10, 8.5) centre (-8.5, 8.5) ccw
  circle A4 centre (0, 0) radius 2.6
  line L6 (2.7393, 3.8) -> (5.5, 6.5607)
  line L7 (5.5, 6.5607) -> (5.5, 8.5)
  line L8 (5.5, 8.5) -> (3.15, 8.5)
  line L9 (3.15, 8.5) -> (3.15, 10)
  line L10 (2.7393, 3.8) -> (-2.7393, 3.8)
  line L11 (-2.7393, 3.8) -> (-5.5, 6.5607)
  line L12 (-5.5, 6.5607) -> (-5.5, 8.5)
  line L13 (-5.5, 8.5) -> (-3.15, 8.5)
  line L14 (-3.15, 8.5) -> (-3.15, 10)
  line L15 (0, 15.5) -> (0, 0)
  line L16 (-8.5, 3.15) -> (-10, 3.15)
  line L17 (-8.5, 5.5) -> (-8.5, 3.15)
  line L18 (-6.5607, 5.5) -> (-8.5, 5.5)
  line L19 (-3.8, 2.7393) -> (-6.5607, 5.5)
  line L20 (-3.8, 2.7393) -> (-3.8, -2.7393)
  line L21 (-3.8, -2.7393) -> (-6.5607, -5.5)
  line L22 (-6.5607, -5.5) -> (-8.5, -5.5)
  line L23 (-8.5, -5.5) -> (-8.5, -3.15)
  line L24 (-8.5, -3.15) -> (-10, -3.15)
  line L25 (-3.15, -8.5) -> (-3.15, -10)
  line L26 (-5.5, -8.5) -> (-3.15, -8.5)
  line L27 (-5.5, -6.5607) -> (-5.5, -8.5)
  line L28 (-2.7393, -3.8) -> (-5.5, -6.5607)
  line L29 (-2.7393, -3.8) -> (2.7393, -3.8)
  line L30 (2.7393, -3.8) -> (5.5, -6.5607)
  line L31 (5.5, -6.5607) -> (5.5, -8.5)
  line L32 (5.5, -8.5) -> (3.15, -8.5)
  line L33 (3.15, -8.5) -> (3.15, -10)
  line L34 (8.5, -3.15) -> (10, -3.15)
  line L35 (8.5, -5.5) -> (8.5, -3.15)
  line L36 (6.5607, -5.5) -> (8.5, -5.5)
  line L37 (3.8, -2.7393) -> (6.5607, -5.5)
  line L38 (3.8, -2.7393) -> (3.8, 2.7393)
  line L39 (3.8, 2.7393) -> (6.5607, 5.5)
  line L40 (6.5607, 5.5) -> (8.5, 5.5)
  line L41 (8.5, 5.5) -> (8.5, 3.15)
  line L42 (8.5, 3.15) -> (10, 3.15)
  dimension "d1" = 20
  dimension "d2" = 1.5
  dimension "d3" = 1.5
  dimension "d4" = 5.2
  dimension "d5" = 0.75
  dimension "d6" = 6.3
  dimension "d7" = 6.2
  dimension "d8" = 11
  dimension "d10" = 360
  dimension "d13" = 1.5
  constraint horizontal L0
  constraint perpendicular L0 L1
  constraint parallel L0 L2
  constraint parallel L1 L3
  constraint coincident L4 A4.centre
  constraint coincident L5 A4.centre
  constraint coincident A4.centre L15.end
  constraint coincident L4.start L0
  constraint coincident L4.start L3
  constraint tangent L0 A0
  constraint tangent L3 A0
  constraint coincident L5.end L3
  constraint coincident L5.end L2
  constraint tangent L3 A1
  constraint tangent L2 A1
  constraint coincident L4.end L1
  constraint coincident L4.end L2
  constraint tangent L1 A2
  constraint tangent L2 A2
  constraint equal A1 A2
  constraint coincident L5.start L1
  constraint coincident L5.start L0
  constraint tangent L1 A3
  constraint tangent L0 A3
  constraint equal A1 A3
  constraint parallel L4 L6
  constraint vertical L7
  constraint perpendicular L7 L8
  constraint coincident L0 L9.end
  constraint perpendicular L0 L9
  constraint horizontal L10
  constraint perpendicular L6 L11
  constraint vertical L12
  constraint perpendicular L12 L13
  constraint coincident L0 L14.end
  constraint perpendicular L0 L14
  constraint equal L6 L11
  constraint vertical L15
  constraint symmetric L9 L14 L15
  constraint symmetric L6 L11 L15
  constraint symmetric L7 L12 L15
  constraint symmetric L8 L13 L15
  measures "d1" distance of L4.start L5.start
  measures "d2" radius of A0
  measures "d3" radius of A1
  measures "d4" diameter of A4
  measures "d5" distance of L4 L6
  measures "d6" distance of L9 L14
  measures "d7" distance of L0 L10
  measures "d8" distance of L7 L12
  measures "d13" distance of L8.end L9.end
extrude "拉伸1" add sketch "草图1" along normal blind 100 contours L0 L1 L2 L3 A0 A1 A2 A3 L6 L7 L8 L9 L10 L11 L12 L13 L14 L16 L17 L18 L19 L20 L21 L22 L23 L24 L25 L26 L27 L28 L29 L30 L31 L32 L33 L34 L35 L36 L37 L38 L39 L40 L41 L42
ref_plane "工作平面1" through (-10, 0, 0) normal (1, 0, 0) x (0, 1, 0)
sketch "草图3" plane through (-10, 0, 0) normal (1, 0, 0) x (0, 1, 0)
  line L0 (0, 0) -> (0, 100)
  dimension "d15" = 100
  constraint vertical L0
  constraint coincident origin L0
  constraint coincident L0.start origin
  measures "d15" distance of L0.start L0.end
sketch "草图4" plane through (0, 0, 0) normal (0, 0, 1) x (1, 0, 0)
sketch "草图5" plane through (0, 0, 100) normal (0, 0, 1) x (-1, 0, 0)
  circle A0 centre (0, 0) radius 2.6
  line L0 (-3.8, 2.7393) -> (-3.8, -2.7393)
  line L1 (-3.8, -2.7393) -> (-6.5607, -5.5)
  line L2 (-6.5607, -5.5) -> (-8.5, -5.5)
  line L3 (-8.5, -5.5) -> (-8.5, -3.15)
  line L4 (-8.5, -3.15) -> (-10, -3.15)
  line L5 (-10, -3.15) -> (-10, -8.5)
  arc A1 (-10, -8.5) -> (-8.5, -10) centre (-8.5, -8.5) ccw
  line L6 (-8.5, -10) -> (-3.15, -10)
  line L7 (-3.15, -10) -> (-3.15, -8.5)
  line L8 (-3.15, -8.5) -> (-5.5, -8.5)
  line L9 (-5.5, -8.5) -> (-5.5, -6.5607)
  line L10 (-5.5, -6.5607) -> (-2.7393, -3.8)
  line L11 (-2.7393, -3.8) -> (2.7393, -3.8)
  line L12 (2.7393, -3.8) -> (5.5, -6.5607)
  line L13 (5.5, -6.5607) -> (5.5, -8.5)
  line L14 (5.5, -8.5) -> (3.15, -8.5)
  line L15 (3.15, -8.5) -> (3.15, -10)
  line L16 (3.15, -10) -> (8.5, -10)
  arc A2 (8.5, -10) -> (10, -8.5) centre (8.5, -8.5) ccw
  line L17 (10, -8.5) -> (10, -3.15)
  line L18 (10, -3.15) -> (8.5, -3.15)
  line L19 (8.5, -3.15) -> (8.5, -5.5)
  line L20 (8.5, -5.5) -> (6.5607, -5.5)
  line L21 (6.5607, -5.5) -> (3.8, -2.7393)
  line L22 (3.8, -2.7393) -> (3.8, 2.7393)
  line L23 (3.8, 2.7393) -> (6.5607, 5.5)
  line L24 (6.5607, 5.5) -> (8.5, 5.5)
  line L25 (8.5, 5.5) -> (8.5, 3.15)
  line L26 (8.5, 3.15) -> (10, 3.15)
  line L27 (10, 3.15) -> (10, 8.5)
  arc A3 (10, 8.5) -> (8.5, 10) centre (8.5, 8.5) ccw
  line L28 (8.5, 10) -> (3.15, 10)
  line L29 (3.15, 10) -> (3.15, 8.5)
  line L30 (3.15, 8.5) -> (5.5, 8.5)
  line L31 (5.5, 8.5) -> (5.5, 6.5607)
  line L32 (5.5, 6.5607) -> (2.7393, 3.8)
  line L33 (2.7393, 3.8) -> (-2.7393, 3.8)
  line L34 (-2.7393, 3.8) -> (-5.5, 6.5607)
  line L35 (-5.5, 6.5607) -> (-5.5, 8.5)
  line L36 (-5.5, 8.5) -> (-3.15, 8.5)
  line L37 (-3.15, 8.5) -> (-3.15, 10)
  line L38 (-3.15, 10) -> (-8.5, 10)
  arc A4 (-8.5, 10) -> (-10, 8.5) centre (-8.5, 8.5) ccw
  line L39 (-10, 8.5) -> (-10, 3.15)
  line L40 (-10, 3.15) -> (-8.5, 3.15)
  line L41 (-8.5, 3.15) -> (-8.5, 5.5)
  line L42 (-8.5, 5.5) -> (-6.5607, 5.5)
  line L43 (-6.5607, 5.5) -> (-3.8, 2.7393)
  constraint coincident A0.centre origin

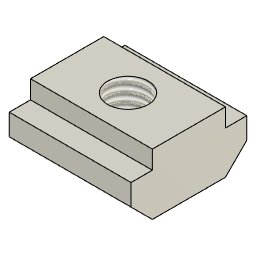
design "20M4_T型滑块"
Autodesk Fusion 360 part; units mm, degrees
sketch "草图1" plane through (0, 0, 0) normal (1, 0, 0) x (0, 1, 0)
  line L0 (0, 80) -> (0, -73.7611) construction
  line L1 (-3, 0) -> (3, 0)
  line L2 (3, 0) -> (3, -1.5)
  line L3 (3, -1.5) -> (4.75, -1.5)
  line L4 (3, -5) -> (-3, -5)
  line L5 (-4.75, -1.5) -> (-3, -1.5)
  line L6 (-3, -1.5) -> (-3, 0)
  line L7 (4.75, -1.5) -> (4.75, -3.25)
  line L8 (4.75, -3.25) -> (3, -5)
  line L9 (-4.75, -1.5) -> (-4.75, -3.25)
  line L10 (-4.75, -3.25) -> (-3, -5)
  dimension "d1" = 6
  dimension "d2" = 6
  dimension "d3" = 1.5
  dimension "d4" = 5
  dimension "d11" = 9.5
  dimension "d12" = 45
  constraint vertical L0
  constraint coincident origin L0
  constraint perpendicular L0 L1
  constraint perpendicular L1 L2
  constraint perpendicular L0 L3
  constraint perpendicular L0 L4
  constraint perpendicular L0 L5
  constraint perpendicular L1 L6
  constraint symmetric L0 L2 L6
  constraint symmetric L0 L3 L5
  constraint perpendicular L3 L7
  constraint perpendicular L5 L9
  constraint symmetric L0 L8 L10
  measures "d1" distance of L4.start L4.end
  measures "d2" distance of L1.start L1.end
  measures "d3" distance of L1.end L2.end
  measures "d4" distance of L1 L4
  measures "d11" distance of L7 L9
  measures "d12" angle of L4 L10
extrude "拉伸1" add sketch "草图1" along normal mid plane 10
sketch "草图2" plane through (0, 0, 0) normal (0, 0, 1) x (1, 0, 0)
  circle A0 centre (0, 0) radius 2.5
  dimension "d7" = 5
  constraint coincident A0.centre origin
  measures "d7" diameter of A0
hole "孔1" at (0, 0, 0) direction (0, 0, -1) diameter 3.332 depth 3 tip angle 180
thread "螺纹1" "ISO Metric profile 4.0 M4x0.7 6H"

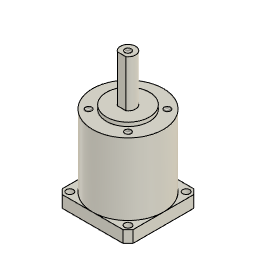
design "Reducer_28*33"
Autodesk Fusion 360 part; units mm, degrees
sketch "草图1" plane through (0, 0, 0) normal (0, 0, 1) x (1, 0, 0)
  line L0 (12, 14) -> (-12, 14)
  line L1 (-14, 12) -> (-14, -12)
  line L2 (-12, -14) -> (12, -14)
  line L3 (14, -12) -> (14, 12)
  line L4 (14, 14) -> (-14, -14) construction
  line L5 (-14, 14) -> (14, -14) construction
  line L6 (12, 14) -> (14, 12)
  line L7 (14, -12) -> (12, -14)
  line L8 (-12, -14) -> (-14, -12)
  line L9 (-14, 12) -> (-12, 14)
  circle A0 centre (-11.5, -11.5) radius 1.4
  circle A1 centre (11.5, -11.5) radius 1.4
  circle A2 centre (11.5, 11.5) radius 1.4
  circle A3 centre (-11.5, 11.5) radius 1.4
  circle A4 centre (0, 0) radius 14
  dimension "d1" = 28
  dimension "d43" = 2
  dimension "d44" = 2
  dimension "d45" = 2
  dimension "d46" = 2
  dimension "d47" = 2
  dimension "d48" = 2
  dimension "d49" = 2
  dimension "d50" = 2
  dimension "d75" = 360
  dimension "d76" = 2.8
  dimension "d77" = 11.5
  dimension "d78" = 11.5
  dimension "d79" = 28
  constraint horizontal L0
  constraint perpendicular L0 L1
  constraint parallel L0 L2
  constraint parallel L1 L3
  constraint coincident L4 A4.centre
  constraint coincident L5 A4.centre
  constraint coincident A4.centre origin
  constraint coincident L4.start L0
  constraint coincident L4.start L3
  constraint coincident L5.end L3
  constraint coincident L5.end L2
  constraint coincident L4.end L2
  constraint coincident L4.end L1
  constraint coincident L5.start L1
  constraint coincident L5.start L0
  measures "d1" distance of L4.start L5.start
  measures "d43" distance of L4.start L0.start
  measures "d44" distance of L4.start L3.end
  measures "d45" distance of L5.end L3.start
  measures "d46" distance of L5.end L2.end
  measures "d47" distance of L4.end L2.start
  measures "d48" distance of L4.end L1.end
  measures "d49" distance of L5.start L1.start
  measures "d50" distance of L5.start L0.end
  measures "d76" diameter of A2
  measures "d77" vertical distance of A4.centre A2.centre
  measures "d78" horizontal distance of A4.centre A2.centre
  measures "d79" diameter of A4
extrude "拉伸1" add sketch "草图1" along normal blind 33 contours L0 L3 L6 A4 | L0 L1 L9 A4 | A4 | L2 L3 L7 A4 | L1 L2 L8 A4 | A0 | A1 | A2 | A3 makes body 1
extrude "拉伸2" cut sketch "草图1" along normal blind 10 contours A0 | A1 | A2 | A3 bodies 1
sketch "草图3" plane through (0, 0, 33) normal (0, 0, 1) x (-1, 0, 0)
  line L0 (-14, 12) -> (-14, -12)
  line L1 (-12, -14) -> (12, -14)
  line L2 (14, -12) -> (14, 12)
  line L3 (12, 14) -> (-12, 14)
  circle A0 centre (0, 0) radius 8.5
  line L4 (-12, 14) -> (-14, 12)
  line L5 (-14, -12) -> (-12, -14)
  line L6 (12, -14) -> (14, -12)
  line L7 (14, 12) -> (12, 14)
  dimension "d12" = 17
  constraint coincident A0.centre origin
  measures "d12" diameter of A0
extrude "拉伸3" add sketch "草图3" along normal blind 1.5 contours A0 bodies 1
extrude "拉伸5" cut sketch "草图1" along normal blind 57 from surface at 4.7 contours L0 L3 L6 A4 | L0 L1 L9 A4 | L2 L3 L7 A4 | L1 L2 L8 A4 | A0 | A1 | A2 | A3 bodies 1
sketch "草图4" plane through (0, 0, 34.5) normal (0, 0, 1) x (-1, 0, 0)
  circle A0 centre (0, 0) radius 8.5
  line L0 (-1.6583, 2.5) -> (1.6583, 2.5)
  arc A1 (-1.6583, 2.5) -> (1.6583, 2.5) centre (0, 0) ccw
  point P0 (0, 3)
  dimension "d15" = 6
  dimension "d83" = 2.5
  constraint coincident A0.centre A1.centre
  measures "d15" diameter of A1
  measures "d83" distance of A0.centre L0
extrude "拉伸4" add sketch "草图4" along normal blind 18.5 contours L0 A1 bodies 1
split "分割1" by plane through (0, 0, 34.5) normal (0, 0, 1) bodies 1 makes body 2 at (-1.8935, -2.3269, 46.8333)
copy_body "实体->零部件1" bodies 2 removing the originals makes body 3 in component "Output_Shaft"
sketch "草图6" plane through (0, 0, 33) normal (0, 0, 1) x (-1, 0, 0)
  circle A0 centre (-7.7782, 7.7782) radius 1.5
  circle A1 centre (-7.7782, -7.7782) radius 1.5
  circle A2 centre (7.7782, -7.7782) radius 1.5
  circle A3 centre (7.7782, 7.7782) radius 1.5
  circle A4 centre (0, 0) radius 8.5
  circle A5 centre (0, 0) radius 14
  line L0 (0, 0) -> (-7.7782, 7.7782) construction
  line L1 (18, 0) -> (-26.2074, 0) construction
  circle A6 centre (0, 0) radius 14
  circle A7 centre (0, 0) radius 8.5
  dimension "d30" = 3
  dimension "d32" = 360
  dimension "d80" = 11
  dimension "d82" = 45
  constraint coincident A4.centre A5.centre
  constraint coincident A0.centre L0.end
  constraint horizontal L1
  constraint coincident A4.centre L1
  measures "d30" diameter of A0
  measures "d80" distance of A4.centre A0.centre
  measures "d82" angle of L0 L1
hole "孔1" at (7.7782, -7.7782, 33) at (7.7782, 7.7782, 33) at (-7.7782, 7.7782, 33) at (-7.7782, -7.7782, 33) direction (0, 0, -1) diameter 2.529 depth 10 tip angle 180 bodies 1
thread "螺纹1" "ISO Metric profile 3.0 M3x0.5 6H" major diameter 3.086 minor diameter 2.529 pitch 0.5 angle 60 resizes the face on face at (-7.7151, -9.0411, 29.6667) on face at (7.8412, -9.0411, 29.6667) on face at (7.8412, 6.5152, 29.6667) on face at (-7.7151, 6.5152, 29.6667) on bodies 1
sketch "草图7" plane through (0, 0, 53) normal (0, 0, 1) x (-1, 0, 0)
  arc A0 (-1.6583, 2.5) -> (1.6583, 2.5) centre (0, 0) ccw
  circle A1 centre (0, 0) radius 1.5
  line L0 (1.6583, 2.5) -> (-1.6583, 2.5)
  dimension "d54" = 3
  constraint concentric A0 A1
  measures "d54" diameter of A1
hole "孔1'" at (0, 0, 53) direction (0, 0, -1) diameter 2.529 depth 10 tip angle 180 bodies 3 in component "Output_Shaft"
thread "螺纹1'" "ISO Metric profile 3.0 M3x0.5 6H" major diameter 3.086 minor diameter 2.529 pitch 0.5 angle 60 resizes the face on face at (0.063, -1.2629, 49.6667) on bodies 3 in component "Output_Shaft"
sketch "草图8" plane through (0, 0, 0) normal (0, 0, 1) x (1, 0, 0)
  line L0 (-1.5, -2) -> (1.5, -2)
  arc A0 (1.5, -2) -> (-1.5, -2) centre (0, 0) ccw
  dimension "d58" = 5
  dimension "d65" = 2
  constraint coincident A0.centre origin
  constraint horizontal L0
  measures "d58" diameter of A0
  measures "d65" distance of A0.centre L0